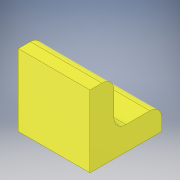
# Autodesk Inventor part: L Filllet
Saved by Autodesk Inventor 2017 SP1 (Build 210196100, 196)
## iProperties
Created: 2016-12-04
Part Number: L Filllet
Material: Generic
Document SubType Name: Modeling
Designer: rbibb
Density: 1 g/cm^3
Appearance: Smooth - Yellow
Author: rbibb
Autodesk Inventor part; units mm, degrees
ref_plane "YZ Plane" through (0, 0, 0) normal (1, 0, 0) x (0, 1, 0)
ref_plane "XZ Plane" through (0, 0, 0) normal (0, 1, 0) x (-1, 0, 0)
ref_plane "XY Plane" through (0, 0, 0) normal (0, 0, 1) x (1, 0, 0)
sketch "Sketch1" plane through (0, 0, 0) normal (1, 0, 0) x (0, 1, 0)
  line L0 (14.8821, 22.5462) -> (-23.2179, 22.5462)
  line L1 (-23.2179, 22.5462) -> (-23.2179, 9.8462)
  line L2 (-23.2179, 9.8462) -> (14.8821, 9.8462)
  line L3 (14.8821, 9.8462) -> (14.8821, 22.5462)
  line L4 (-23.2179, 22.5462) -> (-10.5179, 22.5462)
  line L5 (-10.5179, 22.5462) -> (-10.5179, -15.5538)
  line L6 (-10.5179, -15.5538) -> (-23.2179, -15.5538)
  line L7 (-23.2179, -15.5538) -> (-23.2179, 22.5462)
  point P0 (0, 0)
  dimension "d0" = 38.1
  dimension "d1" = 12.7
  dimension "d2" = 12.7
  dimension "d3" = 38.1
  constraints: 16 end point, 4 parallel, 2 horizontal, 2 perpendicular
  measures "d0" distance of L2.end L1.end
  measures "d1" distance of L1.end L0.end
  measures "d2" distance of L5.end L6.end
  measures "d3" distance of L4.end L5.end
extrude "Extrusion1" add sketch "Sketch1" against normal blind 38.1
fillet "Fillet1" radius 6.35 3 edges at (-19.05, 14.8821, 9.8462) (-19.05, -10.5179, -15.5538) (-19.05, -10.5179, 9.8462)
body "Solid1"
